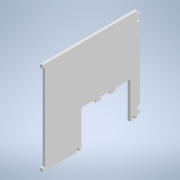
# Autodesk Inventor part: box_right
Saved by Autodesk Inventor 2020 (Build 240168000, 168)
## iProperties
Created: 2020-02-22
Part Number: box_right
Material: Generic
Document SubType Name: Modeling
Designer: Luka
Density: 1 g/cm^3
Appearance: Default
Author: Luka
Autodesk Inventor part; units mm, degrees
ref_plane "YZ Plane" through (0, 0, 0) normal (1, 0, 0) x (0, 1, 0)
ref_plane "XZ Plane" through (0, 0, 0) normal (0, 1, 0) x (-1, 0, 0)
sketch "Sketch1" plane through (0, 0, 0) normal (0, 1, 0) x (-1, 0, 0)
  line L0 (200, 200) -> (0, 200)
  line L1 (0, 200) -> (0, 0)
  line L2 (0, 0) -> (200, 0)
  line L3 (200, 0) -> (200, 200)
  dimension "d0" = 200
  dimension "d1" = 200
  constraints: 8 end point, 2 parallel, 1 horizontal, 1 perpendicular
  measures "d0" distance of L2.end L1.end
  measures "d1" distance of L1.end L0.end
extrude "Extrusion1" add sketch "Sketch1" along normal blind 200
shell "Shell1" thickness 5 removed faces 1 at (-66.6667, 200, 133.3333)
sketch "Sketch2" plane through (-200, 0, 200) normal (0, 0, 1) x (1, 0, 0)
  line L0 (155, 160) -> (158.5, 160)
  line L1 (158.5, 160) -> (158.5, 130)
  line L2 (158.5, 130) -> (155, 130)
  line L3 (155, 130) -> (155, 160)
  line L4 (0, 0) -> (0, 200) projected
  line L5 (200, 0) -> (200, 200) projected
  line L6 (0, 200) -> (200, 200) projected
  line L7 (120, 160) -> (40, 160)
  line L8 (40, 160) -> (40, 125)
  line L9 (40, 125) -> (120, 125)
  line L10 (120, 125) -> (120, 160)
  line L11 (40, 115) -> (120, 115)
  line L12 (120, 115) -> (120, 35)
  line L13 (120, 35) -> (40, 35)
  line L14 (40, 35) -> (40, 115)
  line L15 (69, 25) -> (91, 25)
  line L16 (91, 25) -> (91, 21)
  line L17 (91, 21) -> (69, 21)
  line L18 (69, 21) -> (69, 25)
  line L19 (44, 155) -> (116, 155)
  line L20 (116, 155) -> (116, 130)
  line L21 (116, 130) -> (44, 130)
  line L22 (44, 130) -> (44, 155)
  circle A0 centre (40, 160) radius 5
  circle A1 centre (120, 160) radius 5
  circle A2 centre (120, 125) radius 5
  circle A3 centre (40, 125) radius 5
  line L23 (69, 25) -> (91, 25)
  line L24 (91, 25) -> (91, 35)
  line L25 (91, 35) -> (69, 35)
  line L26 (69, 35) -> (69, 25)
  point P0 (120, 155)
  point P1 (115, 160)
  point P2 (115, 125)
  point P3 (120, 130)
  point P4 (40, 130)
  point P5 (45, 125)
  point P6 (45, 160)
  point P7 (40, 155)
  point P8 (69, 35)
  point P9 (91, 25)
  dimension "COINw" = 3.5
  dimension "COINh" = 30
  dimension "d7" = 155
  dimension "d8" = 41.5
  dimension "d12" = 40
  dimension "d13" = 40
  dimension "LCDw" = 80
  dimension "LCDh" = 35
  dimension "d19" = 22
  dimension "d20" = 4
  dimension "d22" = 29
  dimension "d23" = 10
  dimension "d24" = 10
  dimension "d27" = 72
  dimension "d28" = 25
  dimension "d29" = 4
  dimension "d30" = 4
  dimension "d31" = 5
  dimension "d32" = 5
  dimension "d33" = 10
  dimension "d34" = 10
  dimension "d35" = 10
  constraints: 48 end point, 12 parallel, 7 perpendicular, 6 horizontal, 4 centre point, 4 coincident, 4 collinear, 1 point on line
  measures "COINw" distance of L1.end L2.end
  measures "COINh" distance of L0.end L1.end
  measures "d7" distance between parallel lines of L4 L3
  measures "d8" distance between parallel lines of L5 L1
  measures "d12" distance between parallel lines of L6 L0
  measures "d13" distance between parallel lines of L8 L4
  measures "LCDw" distance between parallel lines of L10 L8
  measures "LCDh" distance between parallel lines of L9 L7
  measures "d19" distance of L15.start L15.end
  measures "d20" distance of L15.end L16.end
  measures "d22" distance from line of L13.end L18
  measures "d23" distance between parallel lines of L15 L13
  measures "d24" distance between parallel lines of L11 L9
  measures "d27" distance of L20.end L21.end
  measures "d28" distance of L19.end L20.end
  measures "d29" distance between parallel lines of L8 L22
  measures "d30" distance between parallel lines of L10 L20
  measures "d31" distance between parallel lines of L7 L19
  measures "d32" distance between parallel lines of L9 L21
  measures "d33" diameter of A0
  measures "d34" diameter of A2
  measures "d35" diameter of A3
extrude "Extrusion2" cut sketch "Sketch2" along normal mid plane 10 contours L0 L1 L2 L3 | L15 L16 L17 L18 | L19 L20 L21 L22
sketch "Sketch3" plane through (0, 0, 200) normal (1, 0, 0) x (0, 0, -1)
  line L0 (0, 0) -> (0, 200) projected
  line L1 (0, 80) -> (200, 80)
  line L2 (0, 0) -> (200, 0) projected
  line L3 (180, 80) -> (180, 0)
  line L4 (80, 80) -> (80, 0)
  line L5 (200, 0) -> (0, 0) projected
  line L6 (5, 5) -> (195, 5) projected
  line L7 (80, 5) -> (195, 5)
  line L8 (200, 0) -> (200, 200) projected
  point P0 (180, 5)
  dimension "d16" = 80
  dimension "d65" = 20
  dimension "d66" = 100
  constraints: 8 end point, 7 point on line, 2 perpendicular, 1 collinear, 1 horizontal
  measures "d16" distance between parallel lines of L2 L1
  measures "d65" distance between parallel lines of L8 L3
  measures "d66" distance between parallel lines of L3 L4
extrude "Extrusion3" cut sketch "Sketch2" against normal blind 2 contours A0 L8 L7 | L7 L8 A0 | L7 A1 L10 A2 L9 A3 L8 A0 | A1 L10 L7 | L7 L10 A1 | A3 L9 L8 | L8 L9 A3 | A2 L9 L10 | L10 L9 A2 | L11 L12 L13 L14 | L13 L24 L15 L26 | L19 L20 L21 L22
hole "Hole1" at (-160, 160, 200) at (-80, 160, 200) at (-80, 125, 200) at (-160, 125, 200) direction (0, 0, -1) diameter 3.5 depth 5
fillet "Fillet2" radius 3 5 edges at (-160, 75, 198) (-80, 75, 198) (-94.5, 35, 198) (-145.5, 35, 198) (-120, 115, 198)
extrude "Extrusion4" cut sketch "Sketch3" against normal blind 5 contours L1 L3 L6 L4
ref_plane "Work Plane3" through (-5, 5, 195) normal (-1, 0, 0) x (0, 0, 1)
split "Split1" plane through (-5, 5, 195) removes the side toward (-1, 0, 0)
sketch "Sketch6" plane through (0, 0, 200) normal (1, 0, 0) x (0, 0, -1)
  line L0 (5, 0) -> (0, 0)
  line L1 (0, 0) -> (0, 200) projected
  line L2 (0, 195) -> (200, 195)
  line L3 (200, 195) -> (200, 200)
  line L4 (0, 200) -> (200, 200) projected
  line L5 (200, 200) -> (0, 200)
  line L6 (0, 200) -> (0, 195)
  line L7 (0, 0) -> (200, 0) projected
  line L8 (0, 0) -> (200, 0)
  line L9 (180, 5) -> (80, 5) projected
  line L10 (200, 5) -> (0, 5)
  line L11 (0, 5) -> (0, 0)
  line L12 (0, 195) -> (0, 189)
  line L13 (0, 189) -> (5, 189)
  line L14 (5, 189) -> (5, 11)
  line L15 (5, 11) -> (0, 11)
  line L16 (0, 11) -> (0, 5)
  line L17 (195, 195) -> (195, 189)
  line L18 (195, 189) -> (200, 189)
  line L19 (200, 189) -> (200, 182)
  line L20 (200, 182) -> (195, 182)
  line L21 (195, 182) -> (195, 174)
  line L22 (195, 174) -> (200, 174)
  line L23 (195, 5) -> (195, 11)
  line L24 (195, 11) -> (200, 11)
  line L25 (200, 0) -> (200, 200) projected
  line L26 (200, 18) -> (195, 18)
  line L27 (195, 18) -> (195, 26)
  line L28 (195, 26) -> (200, 26)
  line L29 (200, 0) -> (200, 200) projected
  line L30 (185, 5) -> (185, 11)
  line L31 (185, 11) -> (190, 11)
  line L32 (190, 11) -> (190, 5)
  line L33 (180, 80) -> (180, 5) projected
  line L34 (75, 5) -> (75, 11)
  line L35 (75, 11) -> (70, 11)
  line L36 (70, 11) -> (70, 5)
  line L37 (80, 5) -> (80, 80) projected
  point P0 (0, 189)
  point P1 (0, 11)
  dimension "d73" = 5
  dimension "d74" = 6
  dimension "d75" = 5
  dimension "d76" = 6
  dimension "d77" = 5
  dimension "d78" = 6
  dimension "d79" = 7
  dimension "d80" = 8
  dimension "d81" = 6
  dimension "d82" = 7
  dimension "d83" = 8
  dimension "d84" = 5
  dimension "d85" = 5
  dimension "d86" = 5
  dimension "d87" = 6
  dimension "d88" = 5
  dimension "d89" = 5
  dimension "d90" = 5
  dimension "d91" = 6
  constraints: 60 end point, 20 perpendicular, 16 point on line, 4 vertical, 3 parallel, 1 horizontal, 5 other
  measures "d73" distance between parallel lines of L4 L2
  measures "d74" distance between parallel lines of L2 L13
  measures "d75" distance between parallel lines of L1 L14
  measures "d76" distance between parallel lines of L15 L10
  measures "d77" distance between parallel lines of L10 L7
  measures "d78" distance between parallel lines of L24 L10
  measures "d79" distance between parallel lines of L26 L24
  measures "d80" distance between parallel lines of L28 L26
  measures "d81" distance between parallel lines of L18 L2
  measures "d82" distance between parallel lines of L20 L18
  measures "d83" distance between parallel lines of L22 L20
  measures "d86" distance of L31.end L30.end
  measures "d87" distance of L30.start L30.end
  measures "d88" distance between parallel lines of L30 L33
  measures "d89" distance of L34.end L35.end
  measures "d90" distance between parallel lines of L37 L34
  measures "d91" distance between parallel lines of L10 L35
extrude "Extrusion11" cut sketch "Sketch6" against normal blind 10 contours L0 L1 L10 L9 L25 L7 | L10 L23 L24 L25 | L1 L13 L14 L15 | L36 L35 L34 L10 | L10 L30 L31 L32 | L26 L27 L28 L25 | L1 L4 L3 L2 | L2 L25 L18 L17 | L22 L21 L20 L25
sketch "Sketch7" plane through (0, 5, 130) normal (0, -1, 0) x (1, 0, 0)
  point P0 (-2.5, 67.5)
hole "Hole2" at (-2.5, 5, 197.5) direction (0, 1, 0) diameter 2 depth 6
sketch "Sketch8" plane through (0, 189, 195) normal (0, -1, 0) x (1, 0, 0)
  line L0 (0, 5) -> (0, 0) projected
  line L1 (-5, 5) -> (0, 5) projected
  point P0 (0, -195)
  point P1 (-2.5, 2.5)
  dimension "d99" = 2.5
  dimension "d100" = 2.5
  measures "d99" distance from line of L0 point (-2.5, 2.5)
  measures "d100" distance from line of L1 point (-2.5, 2.5)
hole "Hole4" at (-2.5, 189, 197.5) direction (0, 1, 0) diameter 2 depth 6
sketch "Sketch9" plane through (0, 189, 5) normal (0, 1, 0) x (1, 0, 0)
  line L0 (-5, 5) -> (0, 5) projected
  line L1 (0, 5) -> (0, 0) projected
  point P0 (-2.5, 2.5)
  dimension "d124" = 2.5
  dimension "d125" = 2.5
  measures "d124" distance from line of L0 point (-2.5, 2.5)
  measures "d125" distance from line of L1 point (-2.5, 2.5)
hole "Hole5" at (-2.5, 189, 2.5) direction (0, -1, 0) diameter 2 depth 7
sketch "Sketch10" plane through (0, 18, 5) normal (0, 1, 0) x (1, 0, 0)
  line L0 (0, 5) -> (0, 0) projected
  line L1 (-5, 5) -> (0, 5) projected
  point P0 (-2.5, 2.5)
  dimension "d115" = 2.5
  dimension "d116" = 2.5
  measures "d115" distance from line of L0 point (-2.5, 2.5)
  measures "d116" distance from line of L1 point (-2.5, 2.5)
hole "Hole6" at (-2.5, 18, 2.5) direction (0, -1, 0) diameter 2 depth 7
sketch "Sketch11" plane through (0, 80, 20) normal (0, -1, 0) x (1, 0, 0)
  line L0 (0, 30) -> (0, 40)
  line L1 (0, 40) -> (-5, 40)
  line L2 (-5, 40) -> (-5, 30)
  line L3 (-5, 30) -> (0, 30)
  line L4 (0, 60) -> (0, 70)
  line L5 (0, 70) -> (-5, 70)
  line L6 (-5, 70) -> (-5, 60)
  line L7 (-5, 60) -> (0, 60)
  line L8 (0, 100) -> (0, 0) projected
  line L9 (-5, 0) -> (-5, 100) projected
  line L10 (0, 100) -> (-5, 100) projected
  line L11 (0, 0) -> (-5, 0) projected
  point P0 (0, -20)
  dimension "d126" = 30
  dimension "d127" = 10
  dimension "d129" = 30
  dimension "d130" = 10
  constraints: 16 end point, 4 collinear, 3 parallel, 1 perpendicular, 1 vertical
  measures "d126" distance between parallel lines of L10 L5
  measures "d127" distance of L5.end L6.end
  measures "d129" distance between parallel lines of L11 L3
  measures "d130" distance between parallel lines of L1 L3
extrude "Extrusion12" add sketch "Sketch11" along normal blind 6 contours L3 L2 L1 L0 | L7 L6 L5 L4
sketch "Sketch12" plane through (0, 80, 50) normal (0, 0, -1) x (-1, 0, 0)
  line L0 (5, -6) -> (0, -6) projected
  line L1 (0, 0) -> (0, -6) projected
  point P0 (0, -80)
  point P1 (2.5, -3)
  dimension "d133" = 3
  dimension "d134" = 2.5
  measures "d133" distance from line of L0 point (2.5, -3)
  measures "d134" distance from line of L1 point (2.5, -3)
hole "Hole7" at (-2.5, 77, 50) direction (0, 0, 1) diameter 2.5 depth 70
equation "\"d45\" = SHELLw"
equation "\"d73\" = SHELLw"
equation "\"d84\" = SHELLw"
equation "\"d85\" = SHELLw"
equation "\"SHELLw\" = 5"
body "Solid1"
